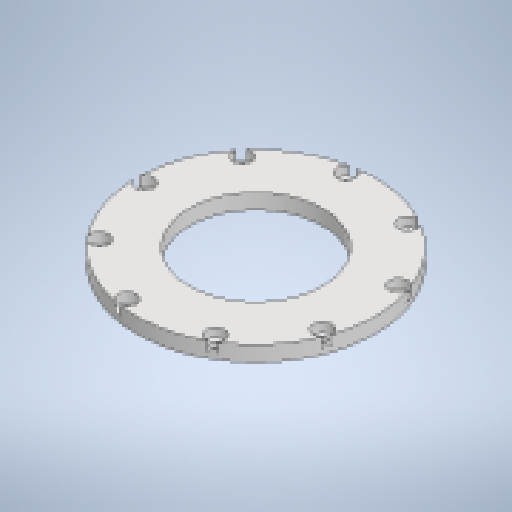
# Autodesk Inventor part: cablepart1
Saved by Autodesk Inventor 2024.3 (Build 283343010, 343A)
## iProperties
Created: 2025-09-27
Part Number: cablepart1
Material: 一般
Document SubType Name: Modeling
Designer: kshau
Density: 1 g/cm^3
Appearance: 既定
Author: kshau
Autodesk Inventor part; units mm, degrees
ref_plane "YZ Plane" through (0, 0, 0) normal (1, 0, 0) x (0, 1, 0)
ref_plane "XZ Plane" through (0, 0, 0) normal (0, 1, 0) x (-1, 0, 0)
ref_plane "XY Plane" through (0, 0, 0) normal (0, 0, 1) x (1, 0, 0)
sketch "スケッチ1" plane through (0, 0, 0) normal (0, 1, 0) x (-1, 0, 0)
  circle A0 centre (0, 0) radius 44.25
  circle A1 centre (0, 0) radius 22
  dimension "d0" = 88.5
  dimension "d3" = 44
  constraints: 2 centre point, 2 coincident
  measures "d0" diameter of A0
  measures "d3" diameter of A1
extrude "押し出し1" add sketch "スケッチ1" along normal blind 5
sketch "スケッチ2" plane through (0, 5, 0) normal (0, 1, 0) x (1, 0, 0)
  circle A0 centre (0, 0) radius 36.5
  point P0 (-36.5, 0)
  point P1 (-27.9606, -23.4617)
  point P2 (-6.3382, -35.9455)
  point P3 (18.25, -31.6099)
  point P4 (34.2988, -12.4837)
  point P5 (34.2988, 12.4837)
  point P6 (18.25, 31.6099)
  point P7 (-6.3382, 35.9455)
  point P8 (-27.9606, 23.4617)
  dimension "d4" = 73
  dimension "d7" = 360
  constraints: 1 coincident, 1 horizontal alignment, 12 other
hole "穴1" at (-36.5, 5, 0) at (-27.9606, 5, 23.4617) at (-6.3382, 5, 35.9455) at (18.25, 5, 31.6099) at (34.2988, 5, 12.4837) at (34.2988, 5, -12.4837) at (18.25, 5, -31.6099) at (-6.3382, 5, -35.9455) at (-27.9606, 5, -23.4617) direction (0, -1, 0) diameter 3.3 end through all
sketch "スケッチ3" plane through (0, 5, 0) normal (0, 1, 0) x (1, 0, 0)
  circle A0 centre (-36.5, 0) radius 1.65 projected
  circle A1 centre (-36.5, 0) radius 3
  circle A2 centre (-27.9606, -23.4617) radius 3
  circle A3 centre (-6.3382, -35.9455) radius 3
  circle A4 centre (18.25, -31.6099) radius 3
  circle A5 centre (34.2988, -12.4837) radius 3
  circle A6 centre (34.2988, 12.4837) radius 3
  circle A7 centre (18.25, 31.6099) radius 3
  circle A8 centre (-6.3382, 35.9455) radius 3
  circle A9 centre (-27.9606, 23.4617) radius 3
  point P0 (0, 0)
  dimension "d16" = 6
  dimension "d19" = 360
  constraints: 9 centre point, 1 coincident, 19 other
  measures "d16" diameter of A1
extrude "押し出し2" cut sketch "スケッチ3" against normal blind 3 contours A0 | A1 | A2 | A3 | A4 | A5 | A6 | A7 | A8 | A9
sketch "スケッチ4" plane through (0, 5, 0) normal (0, 1, 0) x (1, 0, 0)
  circle A0 centre (0, 0) radius 41.75
  circle A1 centre (0, 0) radius 44.25 projected
  line L0 (0, 0) -> (44.25, 0)
  line L1 (44.25, 0) -> (44.25, 4)
  line L2 (44.25, 4) -> (0, 4)
  line L3 (0, 4) -> (0, 0)
  line L4 (44.25, 0) -> (44.25, -4)
  line L5 (44.25, -4) -> (0, -4)
  line L6 (0, -4) -> (0, 0)
  point P0 (44.0688, -4)
  point P1 (41.5579, -4)
  point P2 (41.5579, 4)
  point P3 (44.0688, 4)
  dimension "d23" = 2.5
  dimension "d24" = 4
  constraints: 14 end point, 2 parallel, 2 symmetric about line, 1 centre point, 1 coincident, 1 horizontal, 1 perpendicular, 1 tangent
  measures "d23" radial gap between concentric circles of A1 A0
  measures "d24" distance between parallel lines of L0 L2
extrude "押し出し3" add sketch "スケッチ4" along normal blind 14 contours A0 L5 A1 L2
sketch "スケッチ6" plane through (0, 5, 0) normal (0, 1, 0) x (1, 0, 0)
  circle A0 centre (0, 0) radius 44.25 projected
  line L0 (44.0688, 4) -> (41.5579, 4) projected
  line L1 (44.25, 0) -> (34.25, 0)
  line L2 (34.25, 0) -> (34.25, 4)
  line L3 (34.25, 4) -> (44.25, 4)
  line L4 (44.25, 4) -> (44.25, 0)
  line L5 (44.0688, -4) -> (29.25, -4)
  line L6 (34.25, 0) -> (34.25, -4)
  line L7 (44.25, -4) -> (44.25, 0)
  point P0 (29.25, 4)
  dimension "d31" = 10
  constraints: 14 end point, 4 symmetric about line, 2 parallel, 2 point on line, 1 horizontal, 1 perpendicular, 1 point on circle, 1 tangent
  measures "d31" distance between parallel lines of L4 L2
extrude "押し出し5" cut sketch "スケッチ6" against normal blind 14 contours L1 L2 L3 L0 A0 | A0 L5 L6 L1
sketch "スケッチ7" plane through (0, 5, 0) normal (0, 1, 0) x (1, 0, 0)
  circle A0 centre (0, 0) radius 58
  arc A1 (41.5579, 4) -> (41.5579, -4) centre (0, 0) ccw projected
  circle A2 centre (0, 0) radius 22
  circle A3 centre (0, 0) radius 15
  circle A4 centre (40, 0) radius 18
  circle A5 centre (0, 0) radius 22 projected
  circle A6 centre (0, 0) radius 22 projected
  dimension "d36" = 30
  dimension "d37" = 7
  dimension "d39" = 36
  dimension "d41" = 116
  constraints: 4 centre point, 3 coincident, 3 tangent
  measures "d36" diameter of A3
  measures "d37" radial gap between concentric circles of A3 A2
  measures "d39" diameter of A4
  measures "d41" diameter of A0
